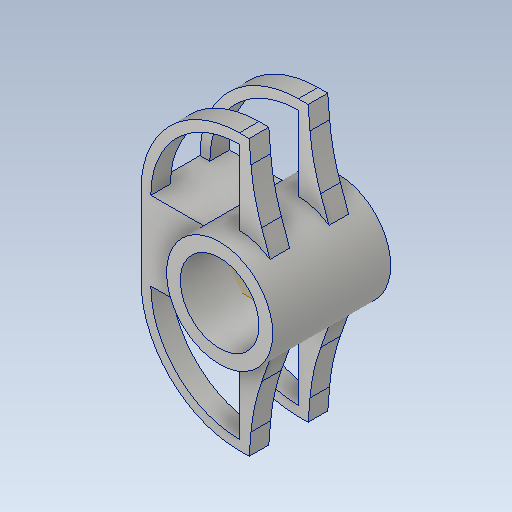
# Autodesk Inventor part: project part
Saved by Autodesk Inventor 2021 (Build 250183000, 183)
## iProperties
Created: 2021-03-09
Part Number: project part
Material: Aluminum 6061
Document SubType Name: Modeling
Designer: Nidhi Upasani
Density: 2.7 g/cm^3
Appearance: Aluminum - Flat
Author: Nidhi Upasani
Autodesk Inventor part; units mm, degrees
ref_plane "YZ Plane" through (0, 0, 0) normal (1, 0, 0) x (0, 1, 0)
ref_plane "XZ Plane" through (0, 0, 0) normal (0, 1, 0) x (-1, 0, 0)
sketch "Sketch1" plane through (0, 0, 0) normal (0, 0, 1) x (1, 0, 0)
  circle A0 centre (0, 0) radius 20
  circle A1 centre (0, 0) radius 27
  line L0 (-27, 0) -> (-50, 0) construction
  line L1 (-50, 20) -> (-50, -20)
  line L2 (-50, 20) -> (-18.1384, 20)
  line L3 (-50, -20) -> (-18.1384, -20)
  dimension "d0" = 40
  dimension "d1" = 54
  dimension "d2" = 23
  dimension "d3" = 50
  dimension "d4" = 40
  dimension "d5" = 20
  dimension "d6" = 20
  constraints: 8 end point, 3 horizontal, 3 point on circle, 2 centre point, 2 coincident, 1 vertical
  measures "d0" diameter of A0
  measures "d1" diameter of A1
  measures "d2" distance of L0.start L0.end
  measures "d3" distance of point (0, 0) L0.end
  measures "d4" distance of L1.start L1.end
  measures "d5" distance of L0.end L1.start
  measures "d6" distance of L1.end L0.end
sketch "Sketch2" plane through (0, 0, 0) normal (0, 0, 1) x (1, 0, 0)
  point P0 (0, 0)
sketch "Sketch3" plane through (0, 0, 0) normal (0, 0, 1) x (1, 0, 0)
  point P0 (0, 0)
extrude "Extrusion1" add sketch "Sketch1" along normal mid plane 40
sketch "Sketch4" plane through (0, 0, 20) normal (0, 0, 1) x (1, 0, 0)
  circle A0 centre (0, 0) radius 20
  circle A1 centre (0, 0) radius 27
  dimension "d9" = 40
  dimension "d10" = 54
  constraints: 2 centre point, 2 coincident
  measures "d9" diameter of A0
  measures "d10" diameter of A1
extrude "Extrusion2" add sketch "Sketch4" along normal blind 10
sketch "Sketch5" plane through (0, 0, -20) normal (0, 0, -1) x (-1, 0, 0)
  circle A0 centre (0, 0) radius 20
  circle A1 centre (0, 0) radius 27
  dimension "d13" = 40
  dimension "d14" = 54
  constraints: 2 centre point, 2 coincident
  measures "d13" diameter of A0
  measures "d14" diameter of A1
extrude "Extrusion3" add sketch "Sketch5" along normal blind 10
sketch "Sketch6" plane through (0, 0, 0) normal (0, 0, 1) x (1, 0, 0)
  point P0 (0, 0)
ref_plane "Work Plane1" through (0, 0, 10) normal (0, 0, 1) x (1, 0, 0)
sketch "Sketch7" plane through (0, 0, 10) normal (0, 0, 1) x (1, 0, 0)
  circle A0 centre (0, 0) radius 20 projected
  line L0 (-50, 20) -> (-18.1384, 20) projected
  arc A1 (0, 70) -> (-50, 20) centre (0, 20) ccw
  arc A2 (0, 65) -> (-45, 20) centre (0, 20) ccw
  line L1 (0, 65) -> (0, 27)
  circle A3 centre (0, 0) radius 27 projected
  line L2 (0, 70) -> (5, 70)
  line L3 (5, 70) -> (5.9668, 58.8209)
  line L4 (11.398, 33.8671) -> (15.6186, 22.0241)
  arc A4 (5.9668, 58.8209) -> (11.398, 33.8671) centre (105.5949, 67.4369) ccw
  point P0 (7.7299, 38.4334)
  point P1 (5, 51.8198)
  dimension "d18" = 50
  dimension "d19" = 45
  dimension "d20" = 38
  dimension "d21" = 5
  dimension "d22" = 5
  dimension "d23" = 31.5666
  dimension "d24" = 94.943
  dimension "d25" = 29.7957
  dimension "d26" = 165.328
  dimension "d27" = 22.1057
  dimension "d28" = 100
  constraints: 8 end point, 8 point on circle, 3 centre point, 3 point on line, 2 tangent, 1 coincident, 1 horizontal, 1 vertical, 1 vertical alignment, 1 other
  measures "d18" radius of A1
  measures "d19" radius of A2
  measures "d20" distance of L1.start L1.end
  measures "d21" distance of L2.start L2.end
  measures "d22" horizontal distance of L1.start L2.end
  measures "d23" vertical distance of L2.end point (7.73, 38.433)
  measures "d24" angle of L3 L2
  measures "d25" vertical distance of point (5, 51.82) L4.end
  measures "d26" angle of L3 L4
  measures "d27" distance from line of point (0, 0) L4
  measures "d28" radius of A4
extrude "Extrusion4" add sketch "Sketch7" along normal blind 10 contours A1 L2 L3 A4 L4 A3 L1 A2 L0
mirror "Mirror1" about plane through (0, 0, 0) normal (0, 0, 1) of "Extrusion4"
mirror "Mirror2" about plane through (0, 0, 0) normal (0, 1, 0) of "Extrusion4", "Mirror1"
scale "Scale1" factors (2, 2, 2) then translate (0, 0, 0) bodies 1
body "Solid1"
